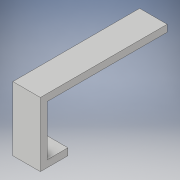
# Autodesk Inventor part: U bracket
Saved by Autodesk Inventor 2019 (Build 230136000, 136)
## iProperties
Created: 2020-10-22
Part Number: U bracket
Material: Generic
Document SubType Name: Modeling
Designer: Delta
Density: 1 g/cm^3
Appearance: Default
Author: Delta
Autodesk Inventor part; units mm, degrees
ref_plane "YZ Plane" through (0, 0, 0) normal (1, 0, 0) x (0, 1, 0)
ref_plane "XZ Plane" through (0, 0, 0) normal (0, 1, 0) x (-1, 0, 0)
ref_plane "XY Plane" through (0, 0, 0) normal (0, 0, 1) x (1, 0, 0)
sketch "Sketch1" plane through (0, 0, 0) normal (1, 0, 0) x (0, 1, 0)
  line L0 (0, 0) -> (3.175, 0)
  line L1 (3.175, 0) -> (3.175, -12.7)
  line L2 (3.175, -12.7) -> (0, -12.7)
  line L3 (0, -12.7) -> (0, 0)
  line L4 (0, 0) -> (29.591, 0)
  line L5 (29.591, 0) -> (29.591, -3.175)
  line L6 (29.591, -3.175) -> (0, -3.175)
  line L7 (0, -3.175) -> (0, 0)
  line L8 (29.591, 0) -> (26.416, 0)
  line L9 (26.416, 0) -> (26.416, -58.42)
  line L10 (26.416, -58.42) -> (29.591, -58.42)
  line L11 (29.591, -58.42) -> (29.591, 0)
  dimension "d0" = 3.175
  dimension "d1" = 12.7
  dimension "d4" = 3.175
  dimension "d5" = 29.591
  dimension "d6" = 3.175
  dimension "d7" = 58.42
  constraints: 24 end point, 6 parallel, 3 horizontal, 3 perpendicular
  measures "d0" distance of L1.end L2.end
  measures "d1" distance of L0.end L1.end
  measures "d4" distance of L9.end L10.end
  measures "d5" distance of L0.start L4.end
  measures "d6" distance between parallel lines of L4 L6
  measures "d7" distance of L10.end L4.end
extrude "Extrusion1" add sketch "Sketch1" along normal blind 12.7
equation "\"d4\" = d0"
equation "\"d6\" = d0"
body "Solid1"
